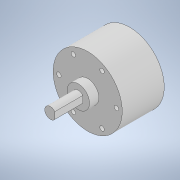
# Autodesk Inventor part: Gearbox
Saved by Autodesk Inventor 2022 (Build 260153000, 153)
## iProperties
Created: 2022-08-13
Part Number: Gearbox
Material: Generic
Document SubType Name: Modeling
Designer: Nick
Density: 3.11078 g/cm^3
Appearance: Default
Mass: 77 g
Surface Area: 59.117 cm^2
Volume: 24.7526 cm^3
Author: Nick
Autodesk Inventor part; units mm, degrees
ref_plane "YZ Plane" through (0, 0, 0) normal (1, 0, 0) x (0, 1, 0)
ref_plane "XZ Plane" through (0, 0, 0) normal (0, 1, 0) x (-1, 0, 0)
ref_plane "XY Plane" through (0, 0, 0) normal (0, 0, 1) x (1, 0, 0)
sketch "Sketch1" plane through (0, 0, 0) normal (0, 0, 1) x (1, 0, 0)
  circle A0 centre (0, 0) radius 18.5
  dimension "d0" = 37
  constraints: 1 centre point, 1 coincident
  measures "d0" diameter of A0
extrude "Extrusion1" add sketch "Sketch1" along normal blind 22.5
sketch "Sketch2" plane through (0, 0, 22.5) normal (0, 0, 1) x (1, 0, 0)
  circle A0 centre (0, 0) radius 6
  dimension "d3" = 12
  constraints: 1 centre point, 1 coincident
  measures "d3" diameter of A0
extrude "Extrusion2" add sketch "Sketch2" along normal blind 5
sketch "Sketch3" plane through (0, 0, 27.5) normal (0, 0, 1) x (1, 0, 0)
  circle A0 centre (0, 0) radius 3
  line L0 (2.4, 1.8) -> (2.4, -1.8)
  line L1 (-3, 1.378) -> (-3, -1.1408) construction
  dimension "d6" = 6
  dimension "d7" = 5.4
  constraints: 4 end point, 2 point on circle, 2 vertical, 1 centre point, 1 coincident, 1 tangent
  measures "d6" diameter of A0
  measures "d7" distance between parallel lines of L0 L1
extrude "Extrusion3" add sketch "Sketch3" along normal blind 15 contours L0 A0 picked at (0.2387, 0.7304)
sketch "Sketch4" plane through (0, 0, 22.5) normal (0, 0, 1) x (1, 0, 0)
  circle A0 centre (-15.415, 0) radius 1.2
  circle A1 centre (15.415, 0) radius 1.2
  arc A2 (2.4, 1.8) -> (2.4, -1.8) centre (0, 0) ccw projected
  line L0 (2.4, -1.8) -> (2.4, 1.8) projected
  circle A3 centre (0, 0) radius 15.415 construction
  dimension "d10" = 30.83
  dimension "d11" = 2.4
  constraints: 3 centre point, 2 horizontal alignment, 2 point on circle, 1 coincident, 1 equal radius
  measures "d10" distance of A1.centre A0.centre
  measures "d11" diameter of A0
extrude "Extrusion4" cut sketch "Sketch4" against normal blind 15 contours A0 | A1
pattern_circular "Circular Pattern1" count 3 over 360 about axis through (0, 0, 0) along (0, 0, 1) of "Extrusion4"
body "Solid1"
